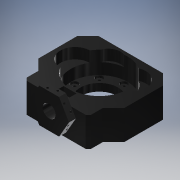
# Autodesk Inventor part: XT-SM-01
Saved by Autodesk Inventor 2017 (Build 210142000, 142)
## iProperties
Created: 2019-11-11
Part Number: XT-SM-01
Material: ABS Plastic
Document SubType Name: Modeling
Designer: Dell
Density: 1.06 g/cm^3
Appearance: Smooth - Black
Author: Dell
Autodesk Inventor part; units mm, degrees
ref_plane "YZ Plane" through (0, 0, 0) normal (1, 0, 0) x (0, 1, 0)
ref_plane "XZ Plane" through (0, 0, 0) normal (0, 1, 0) x (-1, 0, 0)
ref_plane "XY Plane" through (0, 0, 0) normal (0, 0, 1) x (1, 0, 0)
sketch "Sketch1" plane through (0, 0, 0) normal (0, 0, 1) x (1, 0, 0)
  line L0 (-80.1273, -33.5) -> (-80.1273, 39)
  line L1 (80.1273, 39) -> (80.1273, -33.5)
  line L2 (-80.1273, 39) -> (-60.1273, 59)
  line L3 (-60.1273, 59) -> (60.1273, 59)
  line L4 (60.1273, 59) -> (80.1273, 39)
  line L5 (-80.1273, -33.5) -> (-60.1273, -53.5)
  line L6 (-60.1273, -53.5) -> (60.1273, -53.5)
  line L7 (60.1273, -53.5) -> (80.1273, -33.5)
  circle A0 centre (0, 0) radius 35
  point P0 (0, 59)
  point P1 (-80.1273, 2.75)
  dimension "d1" = 160.2547
  dimension "d2" = 72.5
  dimension "d3" = 135
  dimension "d4" = 135
  dimension "d5" = 28.2843
  dimension "d6" = 28.2843
  dimension "d7" = 135
  dimension "d8" = 70
  dimension "d14" = 59
  constraints: 16 end point, 2 horizontal, 2 horizontal alignment, 2 midpoint, 2 vertical, 1 centre point, 1 coincident, 1 perpendicular, 1 vertical alignment
  measures "d1" distance between parallel lines of L1 L0
  measures "d2" distance of L1.start L1.end
  measures "d3" angle of L0 L2
  measures "d4" angle of L1 L4
  measures "d5" distance of L0.end L2.end
  measures "d6" distance of L0.start L5.end
  measures "d7" angle of L0 L5
  measures "d8" diameter of A0
  measures "d14" distance from line of point (0, 0) L3
extrude "Extrusion1" add sketch "Sketch1" along normal blind 55
sketch "Sketch2" plane through (0, 0, 55) normal (0, 0, 1) x (1, 0, 0)
  circle A0 centre (0, 0) radius 53
  dimension "d11" = 106
  constraints: 1 centre point, 1 coincident
  measures "d11" diameter of A0
extrude "Extrusion2" cut sketch "Sketch2" against normal blind 40
sketch "Sketch3" plane through (0, 0, 55) normal (0, 0, 1) x (1, 0, 0)
  arc A0 (-24.527, 52.0056) -> (-13.8164, 9.2419) centre (-14.7916, 31.7208) ccw
  arc A1 (-40.2333, 27.0837) -> (-40.2333, -27.0837) centre (-45, 0) ccw
  arc A2 (47.9099, -7.5429) -> (25.0177, 41.5495) centre (40.7839, 19.0178) ccw
  arc A3 (-24.527, 52.0056) -> (-13.8164, 9.2419) centre (-14.7916, 31.7208) ccw
  circle A4 centre (-14.7916, 31.7208) radius 22.5
  circle A5 centre (40.7839, 19.0178) radius 27.5
  circle A6 centre (-45, 0) radius 27.5
  line L0 (-45, 0) -> (0, 0) construction
  line L1 (0, 0) -> (-14.7916, 31.7208) construction
  line L2 (0, 0) -> (40.7839, 19.0178) construction
  dimension "d15" = 22.5
  dimension "d16" = 27.5
  dimension "d17" = 45
  dimension "d18" = 35
  dimension "d19" = 45
  dimension "d20" = 65
  dimension "d21" = 90
  dimension "d22" = 27.5
  constraints: 8 point on circle, 6 end point, 5 coincident, 4 centre point, 1 horizontal, 9 other
  measures "d15" radius of A0
  measures "d16" radius of A1
  measures "d17" distance of L0.start L0.end
  measures "d18" distance of L0.end L1.end
  measures "d19" distance of L0.end L2.end
  measures "d20" angle of L1 L0
  measures "d21" angle of L2 L1
  measures "d22" radius of A2
extrude "Extrusion3" cut sketch "Sketch3" against normal blind 20
sketch "Sketch4" plane through (0, 0, 15) normal (0, 0, 1) x (1, 0, 0)
  circle A0 centre (46, 0) radius 2.5
  circle A1 centre (32.5269, 32.5269) radius 2.5
  circle A2 centre (0, 46) radius 2.5
  circle A3 centre (-32.5269, 32.5269) radius 2.5
  circle A4 centre (-46, 0) radius 2.5
  circle A5 centre (-32.5269, -32.5269) radius 2.5
  circle A6 centre (0, -46) radius 2.5
  circle A7 centre (32.5269, -32.5269) radius 2.5
  point P0 (0, 0)
  dimension "d25" = 46
  dimension "d26" = 5
  dimension "d29" = 360
  constraints: 8 centre point, 1 horizontal alignment, 17 other
  measures "d25" distance of A0.centre point (0, 0)
  measures "d26" diameter of A0
extrude "Extrusion4" cut sketch "Sketch4" against normal through all
sketch "Sketch6" plane through (0, 0, 55) normal (0, 0, 1) x (1, 0, 0)
  line L0 (-60.1273, -53.5) -> (-80.1273, -33.5) projected
  line L1 (-60.1273, -53.5) -> (60.1273, -53.5)
  line L2 (60.1273, -53.5) -> (60.1273, -80.5)
  line L3 (60.1273, -80.5) -> (-60.1273, -80.5)
  line L4 (-60.1273, -80.5) -> (-60.1273, -53.5)
  point P0 (0, 0)
  dimension "d33" = 27
  constraints: 8 end point, 2 parallel, 1 coincident, 1 horizontal, 1 perpendicular
  measures "d33" distance of L1.end L2.end
extrude "Extrusion5" add sketch "Sketch6" against normal up to surface (55 mm away) from surface at 0
sketch "Sketch7" plane through (0, 0, 15) normal (0, 0, 1) x (1, 0, 0)
  circle A0 centre (46, 0) radius 6.5
  circle A1 centre (46, 0) radius 2.5 projected
  circle A2 centre (32.5269, 32.5269) radius 6.5
  circle A3 centre (0, 46) radius 6.5
  circle A4 centre (-32.5269, 32.5269) radius 6.5
  circle A5 centre (-46, 0) radius 6.5
  circle A6 centre (-32.5269, -32.5269) radius 6.5
  circle A7 centre (0, -46) radius 6.5
  circle A8 centre (32.5269, -32.5269) radius 6.5
  point P0 (0, 0)
  dimension "d36" = 13
  dimension "d39" = 360
  constraints: 8 centre point, 1 coincident, 17 other
  measures "d36" diameter of A0
extrude "Extrusion6" cut sketch "Sketch7" against normal blind 5 contours A0 | A1 | A2 | A3 | A4 | A5 | A6 | A7 | A8
sketch "Sketch8" plane through (0, 0, 15) normal (0, 0, 1) x (1, 0, 0)
  circle A0 centre (0, -46) radius 6.5 projected
  circle A1 centre (-46, 0) radius 6.5 projected
  circle A2 centre (0, 46) radius 6.5 projected
  circle A3 centre (46, 0) radius 6.5 projected
  circle A4 centre (32.5269, 32.5269) radius 6.5 projected
  circle A5 centre (-32.5269, 32.5269) radius 6.5 projected
  circle A6 centre (-32.5269, -32.5269) radius 6.5 projected
  circle A7 centre (32.5269, -32.5269) radius 6.5 projected
  circle A8 centre (0, 0) radius 35 projected
  circle A9 centre (0, 0) radius 53 projected
extrude "Extrusion7" cut sketch "Sketch8" against normal blind 1
sketch "Sketch9" plane through (-60.1273, -80.5, 55) normal (0, -1, 0) x (1, 0, 0)
  line L0 (97.0777, -15) -> (78.6025, -47)
  line L1 (78.6025, -47) -> (41.6521, -47)
  line L2 (41.6521, -47) -> (23.1769, -15)
  line L3 (23.1769, -15) -> (41.6521, 17)
  line L4 (41.6521, 17) -> (78.6025, 17)
  line L5 (78.6025, 17) -> (97.0777, -15)
  line L6 (120.2547, -55) -> (0, -55) projected
  circle A0 centre (60.1273, -15) radius 12
  point P0 (60.1273, -55)
  point P1 (60.1273, -55)
  dimension "d45" = 64
  dimension "d46" = 8
  dimension "d47" = 24
  constraints: 12 end point, 1 centre point, 1 coincident, 1 horizontal, 1 midpoint, 1 vertical alignment, 13 other
  measures "d45" distance between parallel lines of L1 L4
  measures "d46" distance between parallel lines of L6 L1
  measures "d47" diameter of A0
extrude "Extrusion8" add sketch "Sketch9" along normal blind 13
sketch "Sketch10" plane through (-60.1273, -93.5, 55) normal (0, -1, 0) x (1, 0, 0)
  circle A0 centre (60.1273, -15) radius 12 projected
  point P0 (60.1273, -55)
extrude "Extrusion9" cut sketch "Sketch10" against normal blind 39
sketch "Sketch11" plane through (0, 0, 55) normal (0, 0, 1) x (1, 0, 0)
  line L0 (12, -54.5) -> (-12, -54.5) projected
  line L1 (12, -93.5) -> (-12, -93.5) projected
  line L2 (12, -54.5) -> (-12, -54.5)
  line L3 (-12, -54.5) -> (-12, -67.5)
  line L4 (-12, -67.5) -> (12, -67.5)
  line L5 (12, -67.5) -> (12, -54.5)
  line L6 (-12, -54.5) -> (-12, -93.5) projected
  point P0 (0, 0)
  dimension "d52" = 13
  constraints: 8 end point, 2 parallel, 1 horizontal, 1 perpendicular, 1 point on line
  measures "d52" distance of L4.end L0.start
extrude "Extrusion10" cut sketch "Sketch11" against normal blind 15
sketch "Sketch12" plane through (-18.4752, -80.5, 72) normal (0, 0, 1) x (1, 0, 0)
  line L0 (0, -13) -> (0, 0)
  line L1 (36.9504, -13) -> (0, -13)
  line L2 (36.9504, -13) -> (36.9504, 0)
  circle A0 centre (11.4041, -9) radius 2
  circle A1 centre (25.5463, -4) radius 2
  line L3 (11.4041, -9) -> (25.5463, -4) construction
  line L4 (0, 0) -> (36.9504, 0)
  line L5 (0, 0) -> (0, -13) projected
  line L6 (36.9504, -13) -> (0, -13) projected
  point P0 (18.4752, 80.5)
  point P1 (18.4752, -6.5)
  point P2 (18.4752, 0)
  point P3 (0, -6.5)
  point P4 (0, -6.5)
  point P5 (18.4752, -13)
  dimension "d55" = 4
  dimension "d56" = 4
  dimension "d57" = 15
  dimension "d58" = 5
  constraints: 10 end point, 5 midpoint, 2 centre point, 2 horizontal alignment, 2 vertical, 2 vertical alignment, 1 coincident, 1 horizontal
  measures "d55" diameter of A0
  measures "d56" diameter of A1
  measures "d57" distance of L3.start L3.end
  measures "d58" vertical distance of L3.end L3.start
extrude "Extrusion11" cut sketch "Sketch12" against normal blind 20 contours A0 | A1
pattern_circular "Circular Pattern1" count 6 over 360 about axis through (0, -80.5, 40) along (0, -1, 0) of "Extrusion11"
chamfer "Chamfer1" distance 5 angle 45 2 edges at (60.1273, -80.5, 27.5) (-60.1273, -80.5, 27.5)
body "Solid1"
